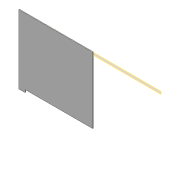
# Autodesk Inventor part: Peça4
Saved by Autodesk Inventor 2020 (Build 240168000, 168)
## iProperties
Created: 2022-07-22
Part Number: Peça4
Material: Genérico
Document SubType Name: Modeling
Designer: gabri
Density: 1 g/cm^3
Appearance: Padrão
Author: gabri
Autodesk Inventor part; units mm, degrees
ref_plane "YZ Plane" through (0, 0, 0) normal (1, 0, 0) x (0, 1, 0)
ref_plane "XZ Plane" through (0, 0, 0) normal (0, 1, 0) x (-1, 0, 0)
ref_plane "XY Plane" through (0, 0, 0) normal (0, 0, 1) x (1, 0, 0)
ref_plane "Plano de trabalho1" through (0, 0, 0) normal (0, 0, 1) x (1, 0, 0)
sketch "Esboço1" plane through (0, 0, 0) normal (0, 0, 1) x (1, 0, 0)
  line L0 (1.7982, -99.874) -> (1.7982, -95.874) projected
  line L1 (1.7982, -99.874) -> (197.7982, -99.874) projected
  line L2 (197.7982, -95.874) -> (197.7982, -99.874) projected
  line L3 (1.7982, -95.874) -> (197.7982, -95.874) projected
  line L4 (-7.8575, 4.6283) -> (104.5488, 4.6283)
  line L5 (104.5488, 4.6283) -> (104.5488, -99.874)
  line L6 (104.5488, -99.874) -> (-7.8575, -99.874)
  line L7 (-7.8575, -99.874) -> (-7.8575, 4.6283)
  point P0 (0, 0)
  point P1 (104.5488, -95.874)
  constraints: 8 end point, 2 parallel, 1 horizontal, 1 perpendicular, 1 point on line
extrude "Extrusão1" add sketch "Esboço1" along normal blind 1 contours L6 L7 L4 L5 L3 L0
